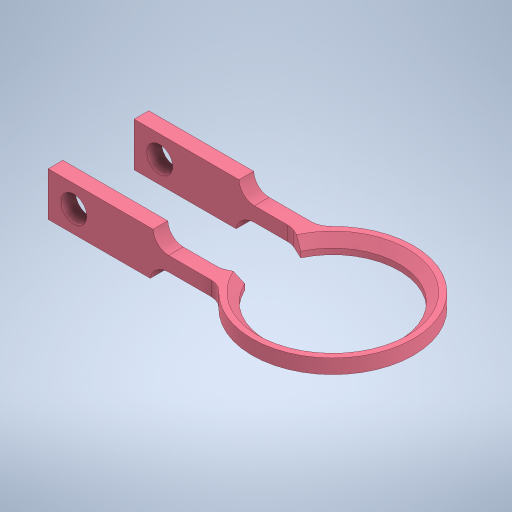
# Autodesk Inventor part: Klemme für SpiegelSlider
Saved by Autodesk Inventor 2023 (Build 270158030, 158C)
## iProperties
Created: 2022-03-08
Part Number: Klemme für SpiegelSlider
Material: Generic
Document SubType Name: Modeling
Designer: XFCM
Density: 1 g/cm^3
Appearance: Default
Author: XFCM
Autodesk Inventor part; units mm, degrees
ref_plane "YZ Plane" through (0, 0, 0) normal (1, 0, 0) x (0, 1, 0)
ref_plane "XZ Plane" through (0, 0, 0) normal (0, 1, 0) x (-1, 0, 0)
sketch "Sketch1" plane through (0, 0, 0) normal (0, 1, 0) x (-1, 0, 0)
  circle A0 centre (0, 0) radius 12.319
  circle A1 centre (0, 0) radius 14
  line L0 (0, 0) -> (12.6883, 5.9167)
  line L1 (0, 0) -> (14, 0) construction
  line L2 (0, 0) -> (12.6883, -5.9167)
  line L3 (0, 0) -> (14, 0) construction
  line L4 (10.6558, 6.1815) -> (40.6558, 6.1815)
  line L5 (40.6558, 6.1815) -> (40.6558, 8.7215)
  line L6 (40.6558, 8.7215) -> (8.7001, 8.7215)
  circle A2 centre (0, 0) radius 11.5
  point P0 (11.1648, -5.2062)
  point P1 (11.1648, 5.2062)
  point P2 (10.9515, 8.7215)
  point P3 (12.5614, 6.1815)
  point P4 (10.4225, -4.8601)
  point P5 (10.4225, 4.8601)
  dimension "d0" = 24.638
  dimension "d1" = 28
  dimension "d2" = 25
  dimension "d3" = 25
  dimension "d6" = 30
  dimension "d7" = 2.54
  dimension "d31" = 23
  constraints: 14 end point, 4 point on circle, 3 centre point, 3 coincident, 3 horizontal, 2 equal length, 2 perpendicular
  measures "d0" diameter of A0
  measures "d1" diameter of A1
  measures "d2" angle of L1 L0
  measures "d3" angle of L2 L3
  measures "d6" distance of L4.start L4.end
  measures "d7" distance of L4.end L5.end
  measures "d31" diameter of A2
extrude "Extrusion1" add sketch "Sketch1" along normal blind 2 contours A0 L0 A2 L2 | L4 A1 L0 A0 | A0 L6 A1 L4 | A0 L2 A1 L6 picked at (8.1725, 8.3931)
extrude "Extrusion2" add sketch "Sketch1" along normal blind 5.08 and the other way blind 2.54 contours A1 L6 L5 L4
sketch "Sketch2" plane through (-40.6558, 5.08, 8.7215) normal (0, 0, 1) x (1, 0, 0)
  line L0 (29.7043, -7.62) -> (0, -7.62) projected
  line L1 (0, -7.62) -> (4.445, -7.62)
  line L2 (4.445, -7.62) -> (4.445, -3.81)
  line L3 (4.445, -3.81) -> (0, -3.81)
  line L4 (0, -3.81) -> (0, -7.62)
  point P0 (40.6558, -5.08)
  point P1 (17.3088, -7.62)
  dimension "d12" = 4.445
  dimension "d13" = 3.81
  constraints: 8 end point, 2 parallel, 1 horizontal, 1 perpendicular
  measures "d12" distance of L3.end L2.end
  measures "d13" distance of L2.end L1.end
hole "Hole1" at (-36.2108, 1.27, 8.7215) direction (0, 0, -1) diameter 4.4958 depth 12.7 tip angle 118 clearance for "Socket Head Cap Screw" size "M4" standard "Ansi Metric M Profile"
ref_plane "Work Plane1" through (0, 0, 0) normal (0, 0, -1) x (-1, 0, 0)
mirror "Mirror1" about plane through (0, 0, 0) normal (0, 0, -1) of "Hole1", "Extrusion2"
sketch "Sketch3" plane through (-10.9515, 5.08, -8.7215) normal (0, 0, -1) x (-1, 0, 0)
  line L0 (0, -7.62) -> (29.7043, -7.62) projected
  line L1 (29.7043, 0) -> (29.7043, -7.62) projected
  line L2 (29.7043, 0) -> (0, 0) projected
  circle A0 centre (25.2593, -3.81) radius 2.2479 projected
  line L3 (0, 0) -> (12, 0)
  line L4 (29.7043, 0) -> (0, 0) projected
  line L5 (12, 0) -> (12, -7.62)
  line L6 (0, -7.62) -> (29.7043, -7.62) projected
  line L7 (1.4361, -5.08) -> (1.4361, -3.08) projected
  line L8 (1.4361, -5.08) -> (12, -5.08)
  line L9 (1.7368, -5.08) -> (1.7368, -3.08) projected
  line L10 (1.7368, -3.08) -> (12, -3.08)
  line L11 (0, -7.62) -> (0, -5.08) projected
  line L12 (0, -3.08) -> (0, 0) projected
  line L13 (0, -5.08) -> (0, -3.08) projected
  line L14 (0, -3.08) -> (0, 0) projected
  line L15 (1.7368, -3.08) -> (0, -3.08)
  line L16 (0, -5.08) -> (0, -3.08) projected
  line L17 (0, -3.08) -> (0, -5.08)
  line L18 (0, -5.08) -> (1.4361, -5.08)
  point P0 (-10.9515, -5.08)
  point P1 (1.7368, -7.62)
  dimension "d22" = 12
  constraints: 14 end point, 5 perpendicular, 4 point on line, 1 collinear
  measures "d22" distance of L2.end L3.end
extrude "Extrusion3" cut sketch "Sketch3" against normal up to surface (17.4431 mm away) contours L11 L18 L8 L5 L0 | L12 L2 L5 L10 L15
fillet "Fillet2" radius 3.175 8 edges at (-12.5614, 1, 6.1815) (-12.5614, 1, -6.1815) (-10.9515, 1, 8.7215) (-10.9515, 1, -8.7215) (-22.9515, 2, -7.4515) (-22.9515, 0, -7.4515) (-22.9515, 0, 7.4515) (-22.9515, 2, 7.4515)
thicken "Thicken1" operation add thickness 0.5 both sides no extend neighbours yes toward (0, 1, 0) faces at (-15.3745, 2, 7.8749)
chamfer "Chamfer2" distance 1.5 angle 45 1 edges at (11.5, 2.5, 0)
body "Solid1"
